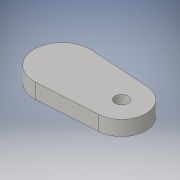
# Autodesk Inventor part: A8-0014
Saved by Autodesk Inventor 2016 SP2 (Build 200236200, 236)
## iProperties
Created: 2017-04-22
Part Number: A8-0014
Material: Generic
Document SubType Name: Modeling
Designer: EV
Density: 1 g/cm^3
Appearance: Default
Author: EV
Autodesk Inventor part; units mm, degrees
ref_plane "YZ Plane" through (0, 0, 0) normal (1, 0, 0) x (0, 1, 0)
ref_plane "XZ Plane" through (0, 0, 0) normal (0, 1, 0) x (-1, 0, 0)
ref_plane "XY Plane" through (0, 0, 0) normal (0, 0, 1) x (1, 0, 0)
sketch "Sketch1" plane through (0, 0, 0) normal (0, 1, 0) x (-1, 0, 0)
  line L0 (0, 0) -> (-16, 0) construction
  line L1 (-0.4688, 7.4853) -> (-16.4063, 6.4873)
  line L2 (-16.4062, -6.4873) -> (-0.4687, -7.4853)
  arc A0 (-0.4687, -7.4853) -> (-0.4688, 7.4853) centre (0, 0) ccw
  arc A1 (-16.4063, 6.4873) -> (-16.4062, -6.4873) centre (-16, 0) ccw
  point P0 (-8, 0)
  point P1 (7.5, 0)
  point P2 (-22.5, 0)
  dimension "d0" = 7.5
  dimension "d1" = 6.5
  dimension "d2" = 30
  constraints: 8 end point, 6 point on circle, 4 tangent, 2 centre point, 1 horizontal, 1 midpoint
  measures "d0" radius of A0
  measures "d1" radius of A1
  measures "d2" distance of point (7.5, 0) point (-22.5, 0)
extrude "Extrusion1" add sketch "Sketch1" along normal blind 4
hole "Hole1" at (16, 4, 0) direction (0, -1, 0) diameter 3.5 end through all
body "Solid1"
